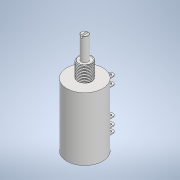
# Autodesk Inventor part: Potenciómetro
Saved by Autodesk Inventor 2022.3 (Build 263350000, 350)
## iProperties
Created: 2023-05-06
Part Number: Potenciómetro
Material: Generic
Document SubType Name: Modeling
Designer: Manuel Hueso Béjar
Density: 1 g/cm^3
Appearance: Default
Author: Manuel Hueso Béjar
Autodesk Inventor part; units mm, degrees
ref_plane "YZ Plane" through (0, 0, 0) normal (1, 0, 0) x (0, 1, 0)
ref_plane "XZ Plane" through (0, 0, 0) normal (0, 1, 0) x (-1, 0, 0)
ref_plane "XY Plane" through (0, 0, 0) normal (0, 0, 1) x (1, 0, 0)
sketch "Sketch1" plane through (0, 0, 0) normal (0, 1, 0) x (-1, 0, 0)
  circle A0 centre (0, 0) radius 10.25
  line L0 (-2.5, -9.25) -> (2.5, -9.25)
  line L1 (2.5, -9.25) -> (2.5, -11.25)
  line L2 (2.5, -11.25) -> (-2.5, -11.25)
  line L3 (-2.5, -11.25) -> (-2.5, -9.25)
  line L4 (-2.5, -9.25) -> (2.5, -11.25) construction
  line L5 (2.5, -9.25) -> (-2.5, -11.25) construction
  point P0 (0, -10.25)
  point P1 (2.5, -9.9404)
  point P2 (-2.5, -9.9404)
  dimension "d0" = 20.5
  dimension "d1" = 5
  dimension "d2" = 2
  constraints: 12 end point, 2 midpoint, 2 parallel, 1 coincident, 1 horizontal, 1 perpendicular, 3 other
  measures "d1" distance of L1.end L2.end
  measures "d2" distance of L0.end L1.end
extrude "Extrusion1" add sketch "Sketch1" along normal blind 36 contours A0 L1 L0 L3 | L3 L0 L1 A0
sketch "Sketch2" plane through (0, 36, 0) normal (0, 1, 0) x (1, 0, 0)
  circle A0 centre (0, 0) radius 4
  dimension "d5" = 8
  constraints: 1 centre point, 1 coincident
  measures "d5" diameter of A0
extrude "Extrusion2" add sketch "Sketch2" along normal blind 9
sketch "Sketch3" plane through (0, 45, 0) normal (0, 1, 0) x (1, 0, 0)
  circle A0 centre (0, 0) radius 2
  dimension "d8" = 4
  constraints: 1 centre point, 1 coincident
  measures "d8" diameter of A0
extrude "Extrusion3" add sketch "Sketch3" along normal blind 13
thread "Thread1" size "M8x0.75" class "6g" standard "ANSI Metric M Profile" full length
sketch "Sketch4" plane through (0, 58, 0) normal (0, 1, 0) x (1, 0, 0)
  line L0 (0.5, -2) -> (-0.5, -2)
  line L1 (-0.5, -2) -> (-0.5, 2)
  line L2 (-0.5, 2) -> (0.5, 2)
  line L3 (0.5, 2) -> (0.5, -2)
  line L4 (0.5, -2) -> (-0.5, 2) construction
  line L5 (-0.5, -2) -> (0.5, 2) construction
  point P0 (0, 0)
  dimension "d13" = 1
  dimension "d14" = 4
  constraints: 12 end point, 2 midpoint, 2 parallel, 1 horizontal, 1 perpendicular
  measures "d13" distance of L1.end L2.end
  measures "d14" distance of L0.end L1.end
extrude "Extrusion4" cut sketch "Sketch4" against normal blind 1.2
fillet "Fillet1" radius 0.2 3 edges at (1.5811, 58, -1.2247) (1.5811, 58, 1.2247) (-2, 58, 0)
extrude "Extrusion5" add sketch "Sketch1" along normal blind 33.5 contours A0 L1 L2 L3
extrude "Extrusion6" cut sketch "Sketch1" along normal blind 2.5 contours A0 L1 L2 L3
sketch "Sketch5" plane through (2.5, 33.5, -11.25) normal (0, 0, -1) x (-1, 0, 0)
  line L0 (0, -31) -> (5, -31) projected
  line L1 (0, -31) -> (5, -31)
  line L2 (5, -31) -> (5, -31.5)
  line L3 (5, -31.5) -> (0, -31.5)
  line L4 (0, -31.5) -> (0, -31)
  line L5 (0, 0) -> (5, 0) projected
  line L6 (0, 0) -> (5, 0)
  line L7 (5, 0) -> (5, -8)
  line L8 (5, -8) -> (0, -8)
  line L9 (0, -8) -> (0, 0)
  line L10 (5, -8) -> (0, -8)
  line L11 (0, -8) -> (0, -7.5)
  line L12 (0, -7.5) -> (5, -7.5)
  line L13 (5, -7.5) -> (5, -8)
  line L14 (0, -8) -> (5, -8)
  line L15 (5, -8) -> (5, -3)
  line L16 (5, -3) -> (0, -3)
  line L17 (0, -3) -> (0, -8)
  line L18 (0, -3) -> (5, -3)
  line L19 (5, -3) -> (5, -3.5)
  line L20 (5, -3.5) -> (0, -3.5)
  line L21 (0, -3.5) -> (0, -3)
  line L22 (5, -31) -> (5, 0) projected
  line L23 (5, -31) -> (0, -31)
  line L24 (0, -31) -> (0, -23)
  line L25 (0, -23) -> (5, -23)
  line L26 (5, -23) -> (5, -31)
  line L27 (0, -23) -> (5, -23)
  line L28 (5, -23) -> (5, -28)
  line L29 (5, -28) -> (0, -28)
  line L30 (0, -28) -> (0, -23)
  line L31 (0, -23) -> (5, -23)
  line L32 (5, -23) -> (5, -23.5)
  line L33 (5, -23.5) -> (0, -23.5)
  line L34 (0, -23.5) -> (0, -23)
  line L35 (5, -28) -> (0, -28)
  line L36 (0, -28) -> (0, -27.5)
  line L37 (0, -27.5) -> (5, -27.5)
  line L38 (5, -27.5) -> (5, -28)
  point P0 (2.5, -33.5)
  point P1 (0, -7.5)
  point P2 (0, -3.5)
  point P3 (5, -3.5)
  point P4 (5, -3)
  point P5 (0, -3)
  dimension "d22" = 5
  dimension "d23" = 0.5
  dimension "d24" = 5
  dimension "d25" = 8
  dimension "d26" = 5
  dimension "d27" = 0.5
  dimension "d28" = 5
  dimension "d29" = 5
  dimension "d30" = 5
  dimension "d31" = 0.5
  dimension "d32" = 5
  dimension "d33" = 8
  dimension "d34" = 5
  dimension "d35" = 5
  dimension "d36" = 5
  dimension "d37" = 0.5
  dimension "d38" = 5
  dimension "d39" = 0.5
  constraints: 72 end point, 18 parallel, 9 horizontal, 9 perpendicular, 1 other
  measures "d22" distance of L2.end L3.end
  measures "d23" distance of L1.end L2.end
  measures "d24" distance of L7.end L8.end
  measures "d25" distance of L6.end L7.end
  measures "d26" distance of L11.end L12.end
  measures "d27" distance of L10.end L11.end
  measures "d28" distance of L16.end L15.end
  measures "d29" distance of L15.end L14.end
  measures "d30" distance of L19.end L20.end
  measures "d31" distance of L18.end L19.end
  measures "d32" distance of L24.end L25.end
  measures "d33" distance of L23.end L24.end
  measures "d34" distance of L28.end L29.end
  measures "d35" distance of L27.end L28.end
  measures "d36" distance of L32.end L33.end
  measures "d37" distance of L31.end L32.end
  measures "d38" distance of L36.end L37.end
  measures "d39" distance of L35.end L36.end
extrude "Extrusion7" add sketch "Sketch5" along normal blind 5 contours L0 L2 L3 L4 | L24 L37 L22 L29 | L24 L25 L22 L33 | L16 L7 L20 L9 | L12 L7 L8 L9
extrude "Extrusion8" add sketch "Sketch5" against normal up to surface contours L0 L2 L3 L4 round surface about axis through (0, 0, 0) along (0, 1, 0) radius 10.25 far side no
sketch "Sketch6" plane through (0, 2, 0) normal (0, -1, 0) x (1, 0, 0)
  line L0 (2.5, -16.25) -> (-2.5, -16.25) projected
  line L1 (0, -16.25) -> (-1.5, -16.25)
  line L2 (0, -16.25) -> (1.5, -16.25) construction
  line L3 (-1.5, -16.25) -> (1.5, -16.25)
  line L4 (1.5, -16.25) -> (1.5, -11.25)
  line L5 (1.5, -11.25) -> (-1.5, -11.25)
  line L6 (-1.5, -11.25) -> (-1.5, -16.25)
  arc A0 (-2.5, -9.9404) -> (2.5, -9.9404) centre (0, 0) ccw projected
  line L7 (2.5, -9.9404) -> (2.5, -11.25)
  line L8 (2.5, -11.25) -> (-2.5, -11.25)
  line L9 (-2.5, -9.9404) -> (-2.5, -16.25) projected
  line L10 (-2.5, -9.9404) -> (-2.5, -11.25)
  line L11 (0, -16.25) -> (0, -15.25)
  line L12 (0, -15.25) -> (0, -13.75)
  circle A1 centre (0, -14.5) radius 0.75
  line L13 (0, -16.25) -> (0, -14.75)
  circle A2 centre (0, -14.75) radius 1.5
  line L14 (1.5, -11.25) -> (1.5, -10.1396)
  line L15 (-1.5, -11.25) -> (-1.5, -10.1396)
  line L16 (2.5, -16.25) -> (-2.5, -16.25)
  line L17 (-2.5, -16.25) -> (-2.5, -11.25)
  line L18 (-2.5, -11.25) -> (2.5, -11.25)
  line L19 (2.5, -11.25) -> (2.5, -16.25)
  point P0 (1.5, -14.75)
  point P1 (-1.5, -14.75)
  dimension "d44" = 1.5
  dimension "d45" = 180
  dimension "d46" = 3
  dimension "d47" = 1
  dimension "d48" = 1.5
  dimension "d49" = 1.5
  constraints: 36 end point, 5 perpendicular, 4 parallel, 3 horizontal, 3 vertical, 2 collinear, 2 midpoint, 2 point on circle, 2 point on line, 1 coincident, 1 vertical alignment, 5 other
  measures "d44" distance of L1.start L1.end
  measures "d45" angle of L1 L2
  measures "d46" distance of L5.end L4.end
  measures "d47" distance of L1.start L11.end
  measures "d48" distance of L11.end L12.end
  measures "d49" distance of L1.start L13.end
extrude "Extrusion9" cut sketch "Sketch6" against normal up to surface (0.5 mm away) contours L8 L14 A0 L7 | L8 L9 A0 L15
extrude "Extrusion10" cut sketch "Sketch6" against normal up to surface (28.5 mm away) contours L0 L4 L8 L19 | L0 A2 L4 | L0 L6 A2 | L0 L9 L8 L6 | A1 L12 | L12 A1
sketch "Sketch7" plane through (0, 0, 0) normal (0, -1, 0) x (1, 0, 0)
  circle A0 centre (0, 0) radius 5
  dimension "d54" = 10
  constraints: 1 centre point, 1 coincident
  measures "d54" diameter of A0
extrude "Extrusion11" add sketch "Sketch7" along normal blind 0.75
fillet "Fillet2" radius 0.75 1 edges at (-5, -0.75, 0)
sketch "Sketch9" plane through (0, 45, 0) normal (1, 0, 0) x (0, 0, 1)
  line L0 (4, 0) -> (4, 9)
  line L1 (4, 9) -> (3.4439, 9)
  line L2 (3.4439, 9) -> (3.4439, 0)
  line L3 (3.4439, 0) -> (4, 0)
  line L4 (0, -24.7515) -> (0, 57.5002) projected
  constraints: 8 end point
revolve "Revolution1" cut sketch "Sketch9" angle 360 about axis through (0, 45, 0) along (0, -1, 0)
sketch "Sketch10" plane through (0, 45, 0) normal (1, 0, 0) x (0, 0, 1)
  line L0 (4, 0) -> (4, 9)
  line L1 (4, 9) -> (3.4439, 9)
  line L2 (3.4439, 9) -> (3.4439, 0)
  line L3 (3.4439, 0) -> (4, 0)
  line L4 (0, -24.7515) -> (0, 57.5002) projected
  constraints: 8 end point
revolve "Revolution2" add sketch "Sketch10" angle 360 about axis through (0, 45, 0) along (0, -1, 0) separate body
sketch "Sketch8" plane through (0, 45, 0) normal (-1, 0, 0) x (0, -1, 0)
  line L0 (-0.4376, -3.482) -> (-0.3751, -3.482) construction
  line L1 (0.0624, -3.9622) -> (-0.0001, -4.0823) construction
  line L2 (-0.7501, -4.0823) -> (-0.8126, -3.9622) construction
  line L3 (-0.3126, -3.482) -> (-0.3751, -3.3619) construction
  line L4 (-0.3751, -3.3619) -> (-0.4376, -3.482) construction
  line L5 (-0.7501, -4.0823) -> (-0.6876, -3.9622) construction
  line L6 (-0.3126, -3.482) -> (-0.0626, -3.9622)
  line L7 (-0.8126, -3.9622) -> (-0.6876, -3.9622) construction
  arc A0 (-0.8126, -3.9622) -> (-0.7501, -4.0002) centre (-0.7501, -3.9297) ccw construction
  line L8 (0.0624, -3.9622) -> (-0.0626, -3.9622) construction
  line L9 (-0.7501, -4.0823) -> (-0.7501, -3.9622) construction
  line L10 (-0.0001, -4.0823) -> (-0.0001, -3.9622) construction
  line L11 (-0.3751, -3.3619) -> (-0.3751, -3.4441) construction
  line L12 (-0.7501, -4.0002) -> (-0.0001, -4.0002)
  arc A1 (-0.7501, -4.0002) -> (-0.6876, -3.9622) centre (-0.7501, -3.9297) ccw
  line L13 (-0.0626, -3.9622) -> (-0.0001, -4.0823) construction
  line L14 (-0.6876, -3.9622) -> (-0.4376, -3.482)
  line L15 (-0.0001, -0.0002) -> (-0.0001, 0.0177)
  line L16 (-0.0001, 0.0177) -> (-0.0001, -0.0002)
  line L17 (-0.0001, -0.0002) -> (0.0334, -0.0002)
  arc A2 (-0.0626, -3.9622) -> (-0.0001, -4.0002) centre (-0.0001, -3.9297) ccw
  arc A3 (-0.0001, -4.0002) -> (0.0624, -3.9622) centre (-0.0001, -3.9297) ccw construction
  arc A4 (-0.3751, -3.4441) -> (-0.4376, -3.482) centre (-0.3751, -3.5145) ccw
  arc A5 (-0.3126, -3.482) -> (-0.3751, -3.4441) centre (-0.3751, -3.5145) ccw
  line L18 (-0.3751, -3.4441) -> (-0.3751, -3.482) construction
  line L19 (-0.3751, -3.482) -> (-0.3126, -3.482) construction
  dimension "d58" = 55
  dimension "d59" = 0.1201
  dimension "d60" = 0.1201
  dimension "Sketch8_ThreadOffset" = 0
  dimension "Sketch8_MajorRadius" = 4
  dimension "d63" = 0.75
  dimension "Sketch8_MinorRadius" = 3.4439
  constraints: 40 end point, 12 point on circle, 10 parallel, 8 tangent, 6 centre point, 6 collinear, 2 midpoint, 2 point on line, 1 horizontal, 1 perpendicular, 3 other
  measures "d58" angle of L6 L14
  measures "d59" distance of L3.end L0.end
  measures "d60" distance of L1.end L10.end
  measures "Sketch8_ThreadOffset" distance between parallel lines of L15 L10
  measures "Sketch8_MajorRadius" distance from line of L12 L15.start
  measures "d63" distance from line of L1.end L9
  measures "Sketch8_MinorRadius" distance edge to line of A5 L17
coil "Coil1" sketch "Sketch8" operation cut axis through (0, 45, 0) along (0, -1, 0) pitch 0.7508 turns 13.986014 hand right bodies 2
equation "\"d58\" = d65"
equation "\"d59\" = 0.160083 * Sketch8_Pitch"
equation "\"d60\" = 0.160083 * Sketch8_Pitch"
equation "\"d63\" = Sketch8_Pitch"
equation "\"d65\" = 55deg"
equation "\"Sketch8_Pitch\" = 0.75"
body "Solid1"
body "Solid2"
